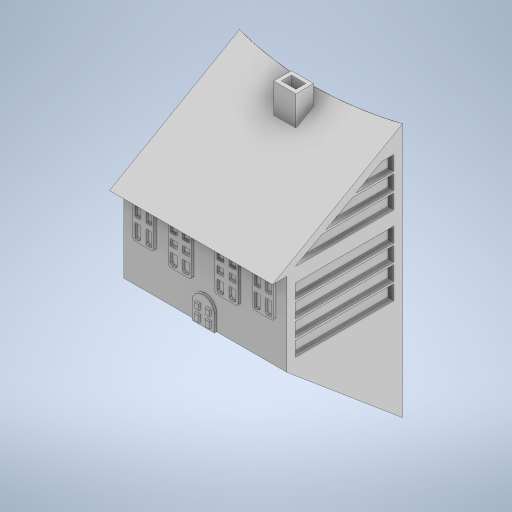
# Autodesk Inventor part: 屋-2 物1
Saved by Autodesk Inventor 2024 (Build 280153000, 153)
## iProperties
Created: 2024-05-21
Part Number: 屋-2 物1
Material: 一般
Document SubType Name: Modeling
Designer: User
Density: 1 g/cm^3
Appearance: 預設
Author: User
Autodesk Inventor part; units mm, degrees
ref_plane "YZ Plane" through (0, 0, 0) normal (1, 0, 0) x (0, 1, 0)
ref_plane "XZ Plane" through (0, 0, 0) normal (0, 1, 0) x (-1, 0, 0)
sketch "草圖1" plane through (0, 0, 0) normal (1, 0, 0) x (0, 1, 0)
  line L0 (0, 0) -> (14.2, 0)
  line L1 (14.2, 0) -> (7.5, 11.7201)
  line L2 (7.5, 11.7201) -> (7.5, 10.4201)
  line L3 (7.5, 10.4201) -> (0, 10.4201)
  line L4 (0, 10.4201) -> (0, 0)
  dimension "d0" = 14.2
  dimension "d1" = 13.5
  dimension "d2" = 1.3
  dimension "d3" = 7.5
  constraints: 10 end point, 2 perpendicular, 1 horizontal, 1 parallel
  measures "d0" distance of L0.start L0.end
  measures "d1" distance of L0.end L1.end
  measures "d2" distance of L1.end L2.end
  measures "d3" distance of L2.end L3.end
extrude "擠出1" add sketch "草圖1" along normal blind 14.7
sketch "草圖2" plane through (0, 0, 0) normal (0, -1, 0) x (1, 0, 0)
  line L0 (6.35, 1.6634) -> (8.35, 1.6634)
  line L1 (8.35, 1.6634) -> (8.35, 3.2634)
  line L2 (8.35, 3.2634) -> (6.35, 3.2634)
  line L3 (6.35, 3.2634) -> (6.35, 1.6634)
  line L4 (14.7, 10.4201) -> (14.7, 0) projected
  line L5 (0, 10.4201) -> (0, 0) projected
  dimension "d6" = 2
  dimension "d7" = 1.6
  dimension "d8" = 6.35
  dimension "d9" = 6.35
  constraints: 8 end point, 2 parallel, 1 horizontal, 1 perpendicular
  measures "d6" distance of L2.end L1.end
  measures "d7" distance of L1.end L0.end
  measures "d8" distance between parallel lines of L4 L1
  measures "d9" distance between parallel lines of L5 L3
extrude "擠出2" add sketch "草圖2" against normal blind 15
sketch "草圖3" plane through (0, 0, 0) normal (-1, 0, 0) x (0, 0, 1)
  line L0 (0.8, 12.1923) -> (0.8, 10.8923)
  line L1 (0.8, 10.8923) -> (4.174, 10.8923)
  line L2 (4.174, 10.8923) -> (1.9, 12.1923)
  line L3 (1.9, 12.1923) -> (0.8, 12.1923)
  line L4 (0.8, 10.6923) -> (4.5239, 10.6923)
  line L5 (0, 14.2) -> (11.7201, 7.5) projected
  line L6 (0.8, 10.6923) -> (0.8, 9.3923)
  line L7 (0.8, 9.3923) -> (6.9097, 9.3923)
  line L8 (6.9097, 9.3923) -> (4.5239, 10.6923)
  line L9 (0.8, 9.1923) -> (0.8, 7.8923)
  line L10 (0.8, 7.8923) -> (9.6625, 7.8923)
  line L11 (9.6625, 7.8923) -> (7.2767, 9.1923)
  line L12 (7.2767, 9.1923) -> (0.8, 9.1923)
  line L13 (0, 0) -> (0, 14.2) projected
  line L14 (0.8, 6.6) -> (9.6625, 6.6)
  line L15 (9.6625, 6.6) -> (9.6625, 5.3)
  line L16 (9.6625, 5.3) -> (0.8, 5.3)
  line L17 (0.8, 5.3) -> (0.8, 6.6)
  line L18 (0.8, 5.1) -> (9.6625, 5.1)
  line L19 (9.6625, 5.1) -> (9.6625, 3.8)
  line L20 (9.6625, 3.8) -> (0.8, 3.8)
  line L21 (0.8, 3.8) -> (0.8, 5.1)
  line L22 (0.8, 3.6) -> (9.6625, 3.6)
  line L23 (9.6625, 3.6) -> (9.6625, 2.3)
  line L24 (9.6625, 2.3) -> (0.8, 2.3)
  line L25 (0.8, 2.3) -> (0.8, 3.6)
  line L26 (0.8, 2.1) -> (9.6625, 2.1)
  line L27 (9.6625, 2.1) -> (9.6625, 0.8)
  line L28 (9.6625, 0.8) -> (0.8, 0.8)
  line L29 (0.8, 0.8) -> (0.8, 2.1)
  line L30 (10.4201, 0) -> (0, 0) projected
  dimension "d12" = 1.3
  dimension "d13" = 1.1
  dimension "d14" = 0.8
  dimension "d15" = 1.3
  dimension "d16" = 1.3
  dimension "d17" = 0.2
  dimension "d18" = 0.2
  dimension "d19" = 0.8
  dimension "d20" = 1.3
  dimension "d21" = 1.3
  dimension "d22" = 1.3
  dimension "d23" = 1.3
  dimension "d24" = 0.2
  dimension "d25" = 0.2
  dimension "d26" = 0.2
  dimension "d27" = 0.8
  constraints: 56 end point, 11 parallel, 10 point on line, 9 perpendicular, 4 horizontal, 1 vertical
  measures "d12" distance between parallel lines of L3 L1
  measures "d13" distance of L2.end L0.start
  measures "d14" distance between parallel lines of L5 L2
  measures "d15" distance between parallel lines of L7 L4
  measures "d16" distance between parallel lines of L10 L12
  measures "d17" distance between parallel lines of L1 L4
  measures "d18" distance between parallel lines of L7 L12
  measures "d19" distance between parallel lines of L13 L0
  measures "d20" distance of L14.end L15.end
  measures "d21" distance of L18.end L19.end
  measures "d22" distance of L22.end L23.end
  measures "d23" distance of L26.end L27.end
  measures "d24" distance between parallel lines of L18 L16
  measures "d25" distance between parallel lines of L22 L20
  measures "d26" distance between parallel lines of L26 L24
  measures "d27" distance between parallel lines of L30 L28
extrude "擠出3" cut sketch "草圖3" against normal blind 0.5
ref_plane "工作平面1" through (7.35, 12.3344, 3.2634) normal (1, 0, 0) x (0, 0, -1)
mirror "鏡射1" about plane through (7.35, 12.3344, 3.2634) normal (1, 0, 0) of "擠出3"
sketch "草圖4" plane through (0, 15, 0) normal (0, 1, 0) x (1, 0, 0)
  line L0 (6.7, -2.0134) -> (8, -2.0134)
  line L1 (8, -2.0134) -> (8, -2.9134)
  line L2 (8, -2.9134) -> (6.7, -2.9134)
  line L3 (6.7, -2.9134) -> (6.7, -2.0134)
  line L4 (8.35, -1.6634) -> (6.35, -1.6634) projected
  line L5 (6.35, -3.2634) -> (8.35, -3.2634) projected
  line L6 (8.35, -3.2634) -> (8.35, -1.6634) projected
  line L7 (6.35, -1.6634) -> (6.35, -3.2634) projected
  point P0 (0, 0)
  dimension "d30" = 0.35
  dimension "d31" = 0.35
  dimension "d32" = 0.35
  dimension "d33" = 0.35
  constraints: 8 end point, 2 parallel, 1 horizontal, 1 perpendicular
  measures "d30" distance between parallel lines of L4 L0
  measures "d31" distance between parallel lines of L5 L2
  measures "d32" distance between parallel lines of L6 L1
  measures "d33" distance between parallel lines of L7 L3
extrude "擠出4" cut sketch "草圖4" against normal blind 10 contours L0 L1 L2 L3
sketch "草圖5" plane through (0, 0, 10.4201) normal (0, 0, 1) x (1, 0, 0)
  line L0 (1.4, 6.8) -> (1.7093, 6.8)
  line L1 (1.7093, 6.6) -> (1.7093, 5.55)
  line L2 (1.7093, 5.55) -> (1.2, 5.55)
  line L3 (1.2, 5.55) -> (1.2, 6.6)
  line L4 (2.7, 6.8) -> (2.2093, 6.8)
  line L5 (2.2093, 6.6) -> (2.2093, 5.55)
  line L6 (2.2093, 5.55) -> (2.7, 5.55)
  line L7 (2.7, 5.55) -> (2.7, 6.6)
  line L8 (1.4, 3.8) -> (1.5093, 3.8)
  line L9 (1.7093, 4) -> (1.7093, 5.05)
  line L10 (1.7093, 5.05) -> (1.2, 5.05)
  line L11 (1.2, 5.05) -> (1.2, 4)
  line L12 (2.5, 3.8) -> (2.4093, 3.8)
  line L13 (2.2093, 4) -> (2.2093, 5.05)
  line L14 (2.2093, 5.05) -> (2.7, 5.05)
  line L15 (2.7, 5.05) -> (2.7, 4)
  line L16 (1.2, 7) -> (2.7, 7)
  line L17 (2.9, 6.8) -> (2.9, 3.8)
  line L18 (2.7, 3.6) -> (1.2, 3.6)
  line L19 (1, 3.8) -> (1, 6.8)
  line L20 (1.2, 3.8) -> (1.2, 5.05)
  line L21 (1.2, 5.55) -> (1.2, 6.8)
  line L22 (1.2, 6.8) -> (1.5093, 6.8)
  line L23 (2.4093, 6.8) -> (2.5, 6.8)
  line L24 (2.7, 6.8) -> (2.7, 5.55)
  line L25 (2.7, 5.05) -> (2.7, 3.8)
  line L26 (2.7, 3.8) -> (2.2093, 3.8)
  line L27 (1.7093, 3.8) -> (1.2, 3.8)
  line L28 (0, 7.5) -> (0, 0) projected
  line L29 (0, 7.5) -> (14.7, 7.5) projected
  arc A0 (1.2, 7) -> (1, 6.8) centre (1.2, 6.8) ccw
  arc A1 (2.9, 6.8) -> (2.7, 7) centre (2.7, 6.8) ccw
  arc A2 (1, 3.8) -> (1.2, 3.6) centre (1.2, 3.8) ccw
  arc A3 (2.7, 3.6) -> (2.9, 3.8) centre (2.7, 3.8) ccw
  arc A4 (1.4, 6.8) -> (1.2, 6.6) centre (1.4, 6.6) ccw
  arc A5 (1.7093, 6.6) -> (1.5093, 6.8) centre (1.5093, 6.6) ccw
  arc A6 (2.4093, 6.8) -> (2.2093, 6.6) centre (2.4093, 6.6) ccw
  arc A7 (2.7, 6.6) -> (2.5, 6.8) centre (2.5, 6.6) ccw
  arc A8 (1.2, 4) -> (1.4, 3.8) centre (1.4, 4) ccw
  arc A9 (1.5093, 3.8) -> (1.7093, 4) centre (1.5093, 4) ccw
  arc A10 (2.2093, 4) -> (2.4093, 3.8) centre (2.4093, 4) ccw
  arc A11 (2.5, 3.8) -> (2.7, 4) centre (2.5, 4) ccw
  line L30 (4.6, 7) -> (4.8, 7)
  line L31 (5, 6.8) -> (5, 5.9)
  line L32 (5, 5.9) -> (4.4, 5.9)
  line L33 (4.4, 5.9) -> (4.4, 6.8)
  line L34 (4.4, 5.4) -> (5, 5.4)
  line L35 (5, 5.4) -> (5, 4.83)
  line L36 (5, 4.83) -> (4.4, 4.83)
  line L37 (4.4, 4.83) -> (4.4, 5.4)
  line L38 (4.4, 4.33) -> (5, 4.33)
  line L39 (5, 4.33) -> (5, 3.53)
  line L40 (4.8, 3.33) -> (4.6, 3.33)
  line L41 (4.4, 3.53) -> (4.4, 4.33)
  line L42 (5.7, 7) -> (5.9, 7)
  line L43 (6.1, 6.8) -> (6.1, 5.9)
  line L44 (6.1, 5.9) -> (5.5, 5.9)
  line L45 (5.5, 5.9) -> (5.5, 6.8)
  line L46 (5.5, 5.4) -> (6.1, 5.4)
  line L47 (6.1, 5.4) -> (6.1, 4.83)
  line L48 (6.1, 4.83) -> (5.5, 4.83)
  line L49 (5.5, 4.83) -> (5.5, 5.4)
  line L50 (5.5, 4.33) -> (6.1, 4.33)
  line L51 (6.1, 4.33) -> (6.1, 3.53)
  line L52 (5.9, 3.33) -> (5.7, 3.33)
  line L53 (5.5, 3.53) -> (5.5, 4.33)
  line L54 (4.4, 7.2) -> (6.1, 7.2)
  line L55 (6.3, 7) -> (6.3, 3.33)
  line L56 (6.1, 3.13) -> (4.4, 3.13)
  line L57 (4.2, 3.33) -> (4.2, 7)
  arc A12 (4.4, 7.2) -> (4.2, 7) centre (4.4, 7) ccw
  arc A13 (4.6, 7) -> (4.4, 6.8) centre (4.6, 6.8) ccw
  arc A14 (5, 6.8) -> (4.8, 7) centre (4.8, 6.8) ccw
  arc A15 (5.7, 7) -> (5.5, 6.8) centre (5.7, 6.8) ccw
  arc A16 (6.1, 6.8) -> (5.9, 7) centre (5.9, 6.8) ccw
  arc A17 (6.3, 7) -> (6.1, 7.2) centre (6.1, 7) ccw
  arc A18 (4.2, 3.33) -> (4.4, 3.13) centre (4.4, 3.33) ccw
  arc A19 (6.1, 3.13) -> (6.3, 3.33) centre (6.1, 3.33) ccw
  arc A20 (5.9, 3.33) -> (6.1, 3.53) centre (5.9, 3.53) ccw
  arc A21 (5.5, 3.53) -> (5.7, 3.33) centre (5.7, 3.53) ccw
  arc A22 (4.8, 3.33) -> (5, 3.53) centre (4.8, 3.53) ccw
  arc A23 (4.4, 3.53) -> (4.6, 3.33) centre (4.6, 3.53) ccw
  point P0 (5, 7)
  point P1 (5, 3.33)
  point P2 (6.1, 3.33)
  dimension "d36" = 1.5
  dimension "d37" = 3
  dimension "d38" = 0.5
  dimension "d39" = 0.5
  dimension "d43" = 0.2
  dimension "d46" = 0.2
  dimension "d47" = 0.2
  dimension "d48" = 0.2
  dimension "d49" = 0.2
  dimension "d50" = 0.2
  dimension "d51" = 0.2
  dimension "d52" = 0.2
  dimension "d53" = 1
  dimension "d54" = 0.5
  dimension "d56" = 0.2
  dimension "d57" = 0.2
  dimension "d58" = 0.6
  dimension "d59" = 1.1
  dimension "d60" = 0.57
  dimension "d61" = 1
  dimension "d62" = 0.5
  dimension "d63" = 0.5
  dimension "d64" = 0.6
  dimension "d65" = 1.1
  dimension "d66" = 0.5
  dimension "d67" = 0.2
  dimension "d68" = 0.2
  dimension "d69" = 0.2
  dimension "d70" = 0.2
  dimension "d71" = 0.2
  dimension "d72" = 1.3
  dimension "d73" = 0.3
  constraints: 112 end point, 48 point on circle, 48 tangent, 36 point on line, 32 parallel, 24 centre point, 21 equal radius, 16 perpendicular, 14 horizontal, 1 collinear
  measures "d36" distance of L25.end L20.start
  measures "d37" distance of L4.start L25.end
  measures "d38" distance between parallel lines of L2 L10
  measures "d39" distance between parallel lines of L5 L1
  measures "d43" distance between parallel lines of L19 L11
  measures "d46" distance between parallel lines of L0 L16
  measures "d47" distance between parallel lines of L4 L16
  measures "d48" distance between parallel lines of L18 L12
  measures "d49" distance between parallel lines of L18 L8
  measures "d50" distance between parallel lines of L17 L7
  measures "d51" distance between parallel lines of L17 L15
  measures "d52" distance between parallel lines of L19 L3
  measures "d53" distance between parallel lines of L28 L19
  measures "d54" distance between parallel lines of L29 L16
  measures "d56" radius of A0
  measures "d57" radius of A4
  measures "d58" distance of L31.end L32.end
  measures "d59" distance of point (5, 7) L31.end
  measures "d60" distance of L34.end L35.end
  measures "d61" distance of L38.end point (5, 3.33)
  measures "d62" distance between parallel lines of L34 L32
  measures "d63" distance between parallel lines of L38 L36
  measures "d64" distance of L43.end L44.end
  measures "d65" distance of point (6.1, 7) L43.end
  measures "d66" distance between parallel lines of L45 L31
  measures "d67" distance between parallel lines of L30 L54
  measures "d68" distance between parallel lines of L55 L43
  measures "d69" distance between parallel lines of L57 L33
  measures "d70" distance between parallel lines of L56 L40
  measures "d71" radius of A12
  measures "d72" distance between parallel lines of L57 L17
  measures "d73" distance between parallel lines of L54 L29
extrude "擠出5" add sketch "草圖5" along normal blind 0.2 contours A4 L21 L22 | L24 A7 L4 | L16 A1 L17 A3 L18 A2 L19 A0 | L54 A17 L55 A19 L56 A18 L57 A12
mirror "鏡射2" about plane through (7.35, 12.3344, 3.2634) normal (1, 0, 0) of "擠出5"
sketch "草圖6" plane through (0, 0, 10.4201) normal (0, 0, 1) x (1, 0, 0)
  line L0 (0, 0) -> (14.7, 0) projected
  line L1 (6.35, 0) -> (8.35, 0)
  line L2 (8.35, 0) -> (8.35, 1.5)
  line L3 (7.35, 2.5) -> (7.35, 2.5)
  line L4 (6.35, 1.5) -> (6.35, 0)
  line L5 (14.7, 7.5) -> (14.7, 0) projected
  line L6 (0, 7.5) -> (0, 0) projected
  arc A0 (7.35, 2.5) -> (6.35, 1.5) centre (7.35, 1.5) ccw
  arc A1 (8.35, 1.5) -> (7.35, 2.5) centre (7.35, 1.5) ccw
  line L7 (6.6429, 0.1687) -> (7.1429, 0.1687)
  line L8 (7.1429, 0.1687) -> (7.1429, 0.8687)
  line L9 (7.1429, 0.8687) -> (6.6429, 0.8687)
  line L10 (6.6429, 0.8687) -> (6.6429, 0.1687)
  line L11 (6.6429, 1.1399) -> (7.1429, 1.1399)
  line L12 (7.1429, 1.1399) -> (7.1429, 1.7399)
  line L13 (7.1429, 1.7399) -> (6.6429, 1.7399)
  line L14 (6.6429, 1.7399) -> (6.6429, 1.1399)
  line L15 (7.6207, 1.7399) -> (8.1207, 1.7399)
  line L16 (8.1207, 1.7399) -> (8.1207, 1.1399)
  line L17 (8.1207, 1.1399) -> (7.6207, 1.1399)
  line L18 (7.6207, 1.1399) -> (7.6207, 1.7399)
  line L19 (7.6207, 0.8687) -> (8.1207, 0.8687)
  line L20 (8.1207, 0.8687) -> (8.1207, 0.1687)
  line L21 (8.1207, 0.1687) -> (7.6207, 0.1687)
  line L22 (7.6207, 0.1687) -> (7.6207, 0.8687)
  point P0 (8.35, 2.5)
  point P1 (6.35, 2.5)
  dimension "d76" = 2
  dimension "d77" = 2.5
  dimension "d78" = 6.35
  dimension "d79" = 6.35
  dimension "d80" = 1
  dimension "d81" = 0.5
  dimension "d82" = 0.7
  dimension "d83" = 0.6
  dimension "d84" = 0.5
  constraints: 40 end point, 10 parallel, 7 point on line, 5 horizontal, 5 perpendicular, 4 point on circle, 4 tangent, 2 centre point, 1 concentric
  measures "d76" distance of point (6.35, 2.5) point (8.35, 2.5)
  measures "d77" distance of point (8.35, 2.5) L1.end
  measures "d78" distance between parallel lines of L5 L2
  measures "d79" distance between parallel lines of L6 L4
  measures "d80" radius of A0
  measures "d81" distance of L9.end L8.end
  measures "d82" distance of L8.end L7.end
  measures "d83" distance of L12.end L11.end
  measures "d84" distance of L16.end L17.end
extrude "擠出6" add sketch "草圖6" along normal blind 0.2 contours L4 A0 A1 L2 L0 | L10 L9 L8 L7 | L14 L13 L12 L11 | L15 L16 L17 L18 | L19 L20 L21 L22
extrude "擠出7" add sketch "草圖6" along normal blind 0.35 draft -10 contours L10 L9 L8 L7 | L14 L13 L12 L11 | L15 L16 L17 L18 | L19 L20 L21 L22
sketch "草圖7" plane through (0, 0, 0) normal (0, -1, 0) x (1, 0, 0)
  line L0 (0, 10.4201) -> (0, 0) projected
  arc A0 (14.7, 0) -> (0, 0) centre (7.35, -39.3189) ccw
  line L1 (14.7, 0) -> (0, 0)
  dimension "d89" = 40
  constraints: 2 end point, 2 point on circle, 1 centre point, 1 horizontal
  measures "d89" radius of A0
extrude "擠出8" cut sketch "草圖7" along normal through all both and the other way through all
sketch "草圖8" plane through (14.7, 0, 0) normal (1, 0, 0) x (0, 0, -1)
  line L0 (-10.4201, 7.5) -> (-10.4201, 0) projected
  line L1 (-10.4201, 0) -> (0, -8.7435)
  line L2 (-10.4201, 0) -> (3.1824, 0) construction
  line L3 (-10.4201, 0) -> (0, 0) projected
  line L4 (0, -8.7435) -> (0, 0)
  dimension "d92" = 40
  constraints: 6 end point, 1 equal length, 1 horizontal, 1 perpendicular
  measures "d92" angle of L1 L2
extrude "擠出9" add sketch "草圖8" against normal up to surface (14.7 mm away)
sketch "草圖9" plane through (7.35, 0, -39.3189) normal (0, 1, 0) x (1, 0, 0)
  line L0 (7.35, -39.3189) -> (7.35, -51.039) projected
  arc A0 (-7.35, -39.3189) -> (7.35, -39.3189) centre (0, 0) ccw
  line L1 (7.35, -39.3189) -> (-7.35, -39.3189)
  constraints: 2 end point, 2 point on circle, 1 centre point, 1 horizontal
extrude "擠出10" cut sketch "草圖9" against normal up to next
